Autodesk Fusion 360 part; units mm, degrees
note: some values were not read from the file. Set by a fixed rule: which sketch regions a step uses.
(part 2 of 3)
  line L698 (-202, 109) -> (-202, 113)
  arc A249 (-204, 107) -> (-202, 109) centre (-204, 109) ccw
  line L699 (-204, 107) -> (-241, 107)
  arc A250 (-241, 107) -> (-243, 105) centre (-241, 105) ccw
  line L700 (-243, 105) -> (-243, 99)
  arc A251 (-245, 97) -> (-243, 99) centre (-245, 99) ccw
  line L701 (-245, 97) -> (-267, 97)
  arc A252 (-332, 126.0001) -> (-330, 124.0001) centre (-330, 126.0001) ccw
  line L702 (-332, 126.0001) -> (-332, 135)
  line L703 (-332, 135) -> (-337, 135)
  line L704 (-337, 135) -> (-337, 133.0001)
  arc A253 (-339, 131.0001) -> (-337, 133.0001) centre (-339, 133.0001) ccw
  arc A254 (-358, 131.0001) -> (-362, 127) centre (-358, 127.0001) ccw
  line L705 (-362, 123) -> (-362, 127)
  arc A255 (-362, 123) -> (-358, 119.0001) centre (-358, 123.0001) ccw
  arc A256 (-337, 117) -> (-339, 119) centre (-339, 117) ccw
  line L706 (-337, 117) -> (-337, 115)
  line L707 (-337, 115) -> (-334, 115)
  arc A257 (-332, 113) -> (-334, 115) centre (-334, 113) ccw
  line L708 (-332, 109) -> (-332, 113)
  arc A258 (-332, 109) -> (-330, 107) centre (-330, 109) ccw
  line L709 (-330, 107) -> (-287, 107)
  arc A259 (-285, 105) -> (-287, 107) centre (-287, 105) ccw
  line L710 (-285, 105) -> (-285, 99)
  arc A260 (-285, 99) -> (-283, 97) centre (-283, 99) ccw
  line L711 (-283, 97) -> (-267, 97)
  line L712 (-267, 124) -> (-330, 124.0001)
  line L713 (-327, 5) -> (-327, 10)
  line L714 (-327, 10) -> (-307, 10)
  arc A261 (-223, 3) -> (-225, 5) centre (-225, 3) ccw
  line L715 (-225, 5) -> (-227, 5)
  line L716 (-227, 5) -> (-227, 10)
  line L717 (-207, 10) -> (-227, 10)
  line L718 (-207, 5) -> (-207, 10)
  line L719 (-207, 5) -> (-209.0021, 5)
  arc A262 (-209.0021, 5) -> (-211.0021, 2.9998) centre (-209.0021, 3) ccw
  line L720 (-211, -15.9146) -> (-211.0021, 2.9998)
  arc A263 (-215, -19.9102) -> (-211, -15.9146) centre (-215, -15.9102) ccw
  line L721 (-219, -19.9102) -> (-215, -19.9102)
  arc A264 (-223, -15.9116) -> (-219, -19.9102) centre (-219, -15.9102) ccw
  line L722 (-223, -15.9116) -> (-223, 3)
  line L723 (-225, 145) -> (-227, 145)
  line L724 (-227, 145) -> (-227, 140)
  line L725 (-207, 140) -> (-227, 140)
  line L726 (-207, 145) -> (-207, 140)
  line L727 (-207, 145) -> (-209.0021, 145)
  arc A265 (-211.0021, 147.0002) -> (-209.0021, 145) centre (-209.0021, 147) ccw
  line L728 (-211.0007, 166.0733) -> (-211.0021, 147.0002)
  arc A266 (-211.0007, 166.0733) -> (-215, 170) centre (-215, 166) ccw
  line L729 (-219, 170) -> (-215, 170)
  arc A267 (-219, 170) -> (-223, 166.0009) centre (-219, 166) ccw
  line L730 (-223, 166.0009) -> (-223, 147)
  arc A268 (-225, 145) -> (-223, 147) centre (-225, 147) ccw
  arc A269 (-311, 147) -> (-309, 145) centre (-309, 147) ccw
  line L731 (-309, 145) -> (-307, 145)
  line L732 (-307, 145) -> (-307, 140)
  line L733 (-327, 140) -> (-307, 140)
  line L734 (-327, 145) -> (-327, 140)
  line L735 (-327, 145) -> (-324.9979, 145)
  arc A270 (-324.9979, 145) -> (-322.9979, 147.0002) centre (-324.9979, 147) ccw
  line L736 (-322.9993, 165.9261) -> (-322.9979, 147.0002)
  arc A271 (-319, 170) -> (-322.9993, 165.9261) centre (-319, 166) ccw
  line L737 (-315, 170) -> (-319, 170)
  arc A272 (-311, 166.0009) -> (-315, 170) centre (-315, 166) ccw
  line L738 (-311, 166.0009) -> (-311, 147)
  circle A273 centre (43.5, 122.75) radius 3
  circle A274 centre (58.5, 122.75) radius 3
  circle A275 centre (73.5, 122.75) radius 3
  circle A276 centre (73.5, 27.25) radius 3
  arc A277 (79.466, 30.6504) -> (82, 35) centre (77, 35) ccw
  circle A278 centre (43.5, 17.25) radius 2.5
  circle A279 centre (58.5, 17.25) radius 2.5
  circle A280 centre (73.5, 132.75) radius 2.5
  circle A281 centre (58.5, 132.75) radius 2.5
  circle A282 centre (43.5, 132.75) radius 2.5
  line L739 (35, 5) -> (35, 10)
  line L740 (57.5, 5) -> (35, 5)
  line L741 (57.5, 10) -> (35, 10)
  line L742 (57.5, 5) -> (80, 5)
  line L743 (80, 5) -> (80, 10)
  line L744 (80, 10) -> (57.5, 10)
  line L745 (-10, -124) -> (-10, -114)
  line L746 (-10, -59) -> (-10, -69)
  line L747 (-13, -74) -> (-12, -74)
  line L748 (-12, -109) -> (-13, -109)
  line L749 (-15, -117) -> (-15, -114)
  arc A283 (-13, -109) -> (-14.3301, -109.5064) centre (-13, -111) ccw
  arc A284 (-12, -109) -> (-10, -107) centre (-12, -107) ccw
  arc A285 (-10, -76) -> (-12, -74) centre (-12, -76) ccw
  line L750 (-10, -76) -> (-10, -80.6987)
  line L751 (-10, -88.0192) -> (-10, -98.0192)
  arc A286 (-15, -72) -> (-14.9997, -72.0383) centre (-13, -72) ccw
  arc A287 (-14.3301, -73.4936) -> (-13, -74) centre (-13, -72) ccw
  line L752 (-15, -72) -> (-15, -67)
  line L753 (-135.6699, -107.8397) -> (-140, -105.3397)
  line L754 (-135.6699, -109.5064) -> (-135.6699, -107.8397)
  arc A288 (-135.6699, -109.5064) -> (-137, -109) centre (-137, -111) ccw
  line L755 (-138, -109) -> (-137, -109)
  line L756 (-140, -105.3398) -> (-140, -107)
  arc A289 (-140, -107) -> (-138, -109) centre (-138, -107) ccw
  line L757 (-139.9897, -75.7973) -> (-140, -80.6987)
  line L758 (-140, -80.6987) -> (-135.6699, -78.1987)
  arc A290 (-137, -74) -> (-135.6699, -73.4936) centre (-137, -72) ccw
  line L759 (-137, -74) -> (-138, -74)
  arc A291 (-138, -74) -> (-140, -76) centre (-138, -76) ccw
  line L760 (-140, -76) -> (-140, -80.6987)
  line L761 (-135.6699, -78.1987) -> (-135.6699, -73.4936)
  arc A292 (-133, -64) -> (-135, -66) centre (-133, -66) ccw
  line L762 (-133, -64) -> (-132, -64)
  arc A293 (-132, -64) -> (-131.6546, -63.9699) centre (-132, -62) ccw
  line L763 (-130.6699, -64.5385) -> (-131.6546, -63.9699)
  line L764 (-130.6699, -69.5385) -> (-130.6699, -64.5385)
  line L765 (-135, -72.0385) -> (-130.6699, -69.5385)
  line L766 (-135.0004, -72.0383) -> (-135, -72.0385)
  arc A294 (-135.0004, -72.0383) -> (-135, -72) centre (-137, -72) ccw
  line L767 (-135, -67) -> (-135, -66)
  line L768 (-135, -72) -> (-135, -67)
  line L769 (-90, -124) -> (-90, -129)
  line L770 (-90, -124) -> (-115, -124)
  line L771 (-115, -124) -> (-115, -129)
  line L772 (-115, -129) -> (-135, -129)
  line L773 (-135, -124) -> (-140, -124)
  line L774 (-140, -124) -> (-140, -114)
  line L775 (-145, -114) -> (-140, -114)
  line L776 (-145, -69) -> (-145, -114)
  line L777 (-140, -69) -> (-145, -69)
  line L778 (-140, -59) -> (-140, -69)
  line L779 (-140, -59) -> (-135, -59)
  line L780 (-135, -54) -> (-135, -59)
  line L781 (-135, -49) -> (-135, -54)
  arc A295 (-131.8566, -44.3575) -> (-135, -49) centre (-130, -49) ccw
  arc A296 (-115, -49) -> (-118.1434, -44.3575) centre (-120, -49) ccw
  line L782 (-115, -54) -> (-115, -49)
  line L783 (-115, -59) -> (-115, -54)
  line L784 (-115, -59) -> (-94.5, -59)
  line L785 (-94.5, -59) -> (-94.5, -39)
  arc A297 (-89.5, -34) -> (-94.5, -39) centre (-89.5, -39) ccw
  line L786 (-135, -129) -> (-135, -124)
  line L787 (-90, -129) -> (-60, -129)
  circle A298 centre (-85, -48) radius 4.075
  circle A299 centre (-275.5, -32.5) radius 4.075
  line L788 (-209.5, -99.5) -> (-209.5, -103.5)
  line L789 (-207.5, -105.5) -> (-206, -105.5)
  line L790 (-204, -103.5) -> (-204, -99.5)
  line L791 (-206, -97.5) -> (-207.5, -97.5)
  arc A300 (-207.5, -97.5) -> (-209.5, -99.5) centre (-207.5, -99.5) ccw
  arc A301 (-204, -99.5) -> (-206, -97.5) centre (-206, -99.5) ccw
  arc A302 (-206, -105.5) -> (-204, -103.5) centre (-206, -103.5) ccw
  arc A303 (-209.5, -103.5) -> (-207.5, -105.5) centre (-207.5, -103.5) ccw
  arc A304 (-321.5, -99.5) -> (-323.5, -97.5) centre (-323.5, -99.5) ccw
  line L792 (-321.5, -99.5) -> (-321.5, -103.5)
  arc A305 (-323.5, -105.5) -> (-321.5, -103.5) centre (-323.5, -103.5) ccw
  line L793 (-323.5, -105.5) -> (-325, -105.5)
  arc A306 (-327, -103.5) -> (-325, -105.5) centre (-325, -103.5) ccw
  line L794 (-327, -103.5) -> (-327, -99.5)
  arc A307 (-325, -97.5) -> (-327, -99.5) centre (-325, -99.5) ccw
  line L795 (-325, -97.5) -> (-323.5, -97.5)
  arc A308 (41.7475, 118.6053) -> (45.2525, 118.6053) centre (43.5, 122.75) ccw
  line L796 (34, 119) -> (39.8003, 119)
  line L797 (47.1997, 119) -> (54.8003, 119)
  arc A309 (56.7475, 118.6053) -> (60.2525, 118.6053) centre (58.5, 122.75) ccw
  line L798 (62.1997, 119) -> (69.8003, 119)
  line L799 (77.1997, 119) -> (81, 119)
  arc A310 (71.7475, 118.6053) -> (75.2525, 118.6053) centre (73.5, 122.75) ccw
  arc A311 (41.7475, 118.6053) -> (39.8003, 119) centre (39.8003, 114) ccw
  arc A312 (47.1997, 119) -> (45.2525, 118.6053) centre (47.1997, 114) ccw
  arc A313 (56.7475, 118.6053) -> (54.8003, 119) centre (54.8003, 114) ccw
  arc A314 (62.1997, 119) -> (60.2525, 118.6053) centre (62.1997, 114) ccw
  arc A315 (71.7475, 118.6053) -> (69.8003, 119) centre (69.8003, 114) ccw
  arc A316 (77.1997, 119) -> (75.2525, 118.6053) centre (77.1997, 114) ccw
  line L800 (-82.0096, -106.5) -> (-77.9904, -106.5)
  line L801 (-72.0096, -106.5) -> (-67.9904, -106.5)
  arc A317 (-289.5, 21) -> (-291.5, 23) centre (-291.5, 21) ccw
  line L802 (-291.5, 23) -> (-327, 23)
  arc A318 (-327, 23) -> (-329, 21) centre (-327, 21) ccw
  line L803 (-329, 15) -> (-329, 21)
  arc A319 (-329, 15) -> (-327, 13) centre (-327, 15) ccw
  line L804 (-249.5, 23) -> (-284.5, 23)
  arc A320 (-284.5, 23) -> (-286.5, 21) centre (-284.5, 21) ccw
  arc A321 (-247.5, 21) -> (-249.5, 23) centre (-249.5, 21) ccw
  line L805 (-337, 108) -> (-337, 94.5)
  arc A322 (-337, 108) -> (-339, 110) centre (-339, 108) ccw
  line L806 (-339, 110) -> (-340, 110)
  arc A323 (-342, 112) -> (-340, 110) centre (-340, 112) ccw
  line L807 (-342, 112) -> (-342, 112.9999)
  arc A324 (-342, 112.9999) -> (-344, 114.9999) centre (-344, 112.9999) ccw
  arc A325 (-366, 122.9999) -> (-358, 114.9999) centre (-358, 122.9999) ccw
  line L808 (-366, 126.9998) -> (-366, 122.9999)
  arc A326 (-358, 134.9998) -> (-366, 126.9998) centre (-358, 126.9998) ccw
  arc A327 (-344, 134.9999) -> (-342, 136.9999) centre (-344, 136.9999) ccw
  line L809 (-342, 136.9999) -> (-342.0001, 145)
  arc A328 (-337, 150) -> (-342.0001, 145) centre (-337, 145) ccw
  line L810 (-337, 150) -> (-329, 150)
  arc A329 (-329, 150) -> (-327, 152) centre (-329, 152) ccw
  line L811 (-327, 166) -> (-327, 152)
  arc A330 (-319, 174) -> (-327, 166) centre (-319, 166) ccw
  line L812 (-315, 174) -> (-319, 174)
  arc A331 (-307, 166.0013) -> (-315, 174) centre (-315, 166) ccw
  line L813 (-307, 152) -> (-307, 166.0013)
  arc A332 (-307, 152) -> (-305, 150) centre (-305, 152) ccw
  line L814 (-305, 150) -> (-304, 150)
  arc A333 (-302, 148) -> (-304, 150) centre (-304, 148) ccw
  line L815 (-302, 147) -> (-302, 148)
  arc A334 (-302, 147) -> (-300, 145) centre (-300, 147) ccw
  line L816 (-300, 145) -> (-286.5, 145)
  line L817 (-247.5, 144.9999) -> (-233.9999, 144.9999)
  arc A335 (-233.9999, 144.9999) -> (-231.9997, 147.0001) centre (-233.9999, 147.0001) ccw
  line L818 (-231.9997, 147.0001) -> (-231.9997, 147.9994)
  arc A336 (-229.999, 150.0001) -> (-231.9997, 147.9994) centre (-229.999, 147.9994) ccw
  line L819 (-229, 150.0001) -> (-229.999, 150.0001)
  arc A337 (-229, 150.0001) -> (-227, 152.0001) centre (-229, 152.0001) ccw
  line L820 (-227, 152.0001) -> (-227, 166.002)
  arc A338 (-219, 174) -> (-227, 166.002) centre (-219, 166) ccw
  line L821 (-219, 174) -> (-215, 174)
  arc A339 (-207, 166) -> (-215, 174) centre (-215, 166) ccw
  line L822 (-207, 166) -> (-207, 152.0001)
  arc A340 (-207, 152.0001) -> (-205, 150.0001) centre (-205, 152.0001) ccw
  line L823 (-197, 150.0001) -> (-205, 150.0001)
  arc A341 (-192, 145.0001) -> (-197, 150.0001) centre (-197, 145.0001) ccw
  line L824 (-192, 145.0001) -> (-192, 136.9999)
  arc A342 (-192, 136.9999) -> (-190, 134.9999) centre (-190, 136.9999) ccw
  arc A343 (-168, 126.9998) -> (-175.9914, 134.9998) centre (-176, 126.9998) ccw
  line L825 (-168, 126.9998) -> (-168, 122.9999)
  arc A344 (-176, 114.9999) -> (-168, 122.9999) centre (-176, 122.9999) ccw
  arc A345 (-190, 114.9999) -> (-192, 112.9999) centre (-190, 112.9999) ccw
  line L826 (-192, 112) -> (-192, 112.9999)
  arc A346 (-194, 110) -> (-192, 112) centre (-194, 112) ccw
  line L827 (-195, 110) -> (-194, 110)
  arc A347 (-195, 110) -> (-197, 108) centre (-195, 108) ccw
  line L828 (-197, 108) -> (-197, 90)
  line L829 (-197, 90) -> (-202, 90)
  line L830 (-202, 90) -> (-202, 75)
  line L831 (-104, 5) -> (-86, 5)
  line L832 (-56, 5) -> (-38, 5)
  line L833 (-104, 145) -> (-86, 145)
  line L834 (-56, 145) -> (-38, 145)
  line L835 (-141, 90) -> (-141, 108)
  line L836 (-141, 60) -> (-141, 42)
  line L837 (-302, 8) -> (-291.5, 8)
  line L838 (-327, 13) -> (-306, 13)
  line L839 (-304, 11) -> (-304, 10)
  line L840 (-289.5, 21) -> (-289.5, 10)
  arc A348 (-304, 11) -> (-306, 13) centre (-306, 11) ccw
  arc A349 (-304, 10) -> (-302, 8) centre (-302, 10) ccw
  arc A350 (-291.5, 8) -> (-289.5, 10) centre (-291.5, 10) ccw
  arc A351 (-244.5001, 10) -> (-242.5001, 8) centre (-242.5001, 10) ccw
  line L841 (-232.0001, 7.9999) -> (-242.5001, 8)
  arc A352 (-232.0001, 7.9999) -> (-230.0001, 9.9999) centre (-232.0001, 9.9999) ccw
  line L842 (-230.0001, 10.9999) -> (-230.0001, 9.9999)
  arc A353 (-228.0001, 12.9999) -> (-230.0001, 10.9999) centre (-228.0001, 10.9999) ccw
  line L843 (-207.0001, 12.9999) -> (-228.0001, 12.9999)
  arc A354 (-207.0001, 12.9999) -> (-205.0001, 14.9999) centre (-207.0001, 14.9999) ccw
  line L844 (-205.0001, 14.9999) -> (-205.0001, 20.9999)
  arc A355 (-205.0001, 20.9999) -> (-207.0001, 22.9999) centre (-207.0001, 20.9999) ccw
  line L845 (-242.4962, 23) -> (-207.0001, 22.9999)
  arc A356 (-242.4962, 23) -> (-244.5001, 21) centre (-242.5001, 21) ccw
  line L846 (-244.5001, 21) -> (-244.5001, 10)
  line L847 (-329, 135) -> (-329, 129)
  arc A357 (-327, 137) -> (-329, 135) centre (-327, 135) ccw
  line L848 (-327, 137) -> (-306, 137)
  arc A358 (-306, 137) -> (-304, 139) centre (-306, 139) ccw
  line L849 (-304, 139) -> (-304, 140)
  arc A359 (-302, 142) -> (-304, 140) centre (-302, 140) ccw
  line L850 (-302, 142) -> (-291.5, 142)
  arc A360 (-289.5, 140) -> (-291.5, 142) centre (-291.5, 140) ccw
  line L851 (-289.5, 129) -> (-289.5, 140)
  arc A361 (-291.5, 127) -> (-289.5, 129) centre (-291.5, 129) ccw
  line L852 (-291.5, 127) -> (-327, 127)
  arc A362 (-329, 129) -> (-327, 127) centre (-327, 129) ccw
  arc A363 (-207.0001, 127.0001) -> (-205.0001, 129.0001) centre (-207.0001, 129.0001) ccw
  line L853 (-205.0001, 135.0001) -> (-205.0001, 129.0001)
  arc A364 (-205.0001, 135.0001) -> (-207.0001, 137.0001) centre (-207.0001, 135.0001) ccw
  line L854 (-207.0001, 137.0001) -> (-228.0001, 137.0001)
  arc A365 (-230.0001, 139.0001) -> (-228.0001, 137.0001) centre (-228.0001, 139.0001) ccw
  line L855 (-230.0001, 139.0001) -> (-230.0001, 140.0001)
  arc A366 (-230.0001, 140.0001) -> (-232.0001, 142.0001) centre (-232.0001, 140.0001) ccw
  line L856 (-232.0001, 142.0001) -> (-242.5001, 142)
  arc A367 (-242.5001, 142) -> (-244.5001, 140) centre (-242.5001, 140) ccw
  line L857 (-244.5001, 129) -> (-244.5001, 140)
  arc A368 (-244.5001, 129) -> (-242.4962, 127) centre (-242.5001, 129) ccw
  line L858 (-242.4962, 127) -> (-207.0001, 127.0001)
  line L859 (-200.5, -98.5) -> (-200.5, -53.5)
  line L860 (-335.5, -76) -> (-335.5, -53.5)
  line L861 (-335.5, -76) -> (-335.5, -98.5)
  line L862 (-335.5, -98.5) -> (-330.5, -98.5)
  line L863 (-330.5, -98.5) -> (-330.5, -53.5)
  line L864 (-335.5, -53.5) -> (-330.5, -53.5)
  line L865 (-136, 10) -> (-141, 10)
  line L866 (-141, 5) -> (-136, 5)
  line L867 (-136, 5) -> (-136, 10)
  line L868 (-141, 10) -> (-141, 5)
  line L869 (-1, 5) -> (-6, 5)
  line L870 (-6, 5) -> (-6, 10)
  line L871 (-6, 10) -> (-1, 10)
  line L872 (-1, 10) -> (-1, 5)
  line L873 (-136, 145) -> (-136, 140)
  line L874 (-136, 140) -> (-141, 140)
  line L875 (-141, 140) -> (-141, 145)
  line L876 (-141, 145) -> (-136, 145)
  line L877 (-6, 145) -> (-6, 140)
  line L878 (-6, 140) -> (-1, 140)
  line L879 (-1, 140) -> (-1, 145)
  line L880 (-1, 145) -> (-6, 145)
  circle A369 centre (-125, -40) radius 2.5
  arc A370 (-119.3006, -41.8753) -> (-130.6994, -41.8753) centre (-125, -40) ccw
  arc A371 (-119.3006, -41.8753) -> (-118.1434, -44.3575) centre (-117.4008, -42.5004) ccw
  arc A372 (-131.8566, -44.3575) -> (-130.6994, -41.8753) centre (-132.5992, -42.5004) ccw
  arc A373 (-15, -49) -> (-18.1435, -44.3575) centre (-20, -49) ccw
  arc A374 (-19.3006, -41.8753) -> (-18.1435, -44.3575) centre (-17.4008, -42.5004) ccw
  arc A375 (-19.3006, -41.8753) -> (-30.6994, -41.8753) centre (-25, -40) ccw
  circle A376 centre (-25, -40) radius 2.5
  arc A377 (-31.8566, -44.3575) -> (-35, -49) centre (-30, -49) ccw
  arc A378 (-31.8566, -44.3575) -> (-30.6994, -41.8753) centre (-32.5992, -42.5004) ccw
  line L881 (-286.5, 5) -> (-286.5, 11)
  line L882 (-284.5, 13) -> (-249.5, 13)
  line L883 (-247.5, 11) -> (-247.5, 5.0001)
  arc A379 (-249.5, 16) -> (-247.5, 18) centre (-249.5, 18) ccw
  line L884 (-249.5, 16) -> (-284.5, 16)
  arc A380 (-286.5, 18) -> (-284.5, 16) centre (-284.5, 18) ccw
  arc A381 (-284.5, 13) -> (-286.5, 11) centre (-284.5, 11) ccw
  arc A382 (-247.5, 11) -> (-249.5, 13) centre (-249.5, 11) ccw
  line L885 (-286.5, 18) -> (-286.5, 21)
  line L886 (-247.5, 21) -> (-247.5, 18)
  line L887 (-284.5, 137) -> (-249.5, 137)
  arc A383 (-284.5, 134) -> (-286.5, 132) centre (-284.5, 132) ccw
  line L888 (-286.5, 132) -> (-286.5, 129)
  arc A384 (-286.5, 129) -> (-284.5, 127) centre (-284.5, 129) ccw
  line L889 (-249.5, 127) -> (-284.5, 127)
  arc A385 (-249.5, 127) -> (-247.5, 129) centre (-249.5, 129) ccw
  line L890 (-247.5, 129) -> (-247.5, 132)
  arc A386 (-247.5, 132) -> (-249.5, 134) centre (-249.5, 132) ccw
  line L891 (-249.5, 134) -> (-284.5, 134)
  arc A387 (-286.5, 139) -> (-284.5, 137) centre (-284.5, 139) ccw
  line L892 (-286.5, 145) -> (-286.5, 139)
  line L893 (-247.5, 139) -> (-247.5, 144.9999)
  arc A388 (-249.5, 137) -> (-247.5, 139) centre (-249.5, 139) ccw
  line L894 (-337, 94.5) -> (-331, 94.5)
  line L895 (-337, 55.5) -> (-331, 55.5)
  line L896 (-329, 92.5) -> (-329, 57.5)
  arc A389 (-329, 92.5) -> (-331, 94.5) centre (-331, 92.5) ccw
  arc A390 (-331, 55.5) -> (-329, 57.5) centre (-331, 57.5) ccw
  arc A391 (76.1918, 30.8561) -> (70.8974, 30.9211) centre (73.5, 27.25) ccw
  line L897 (38, 30) -> (68.0057, 30)
  arc A392 (68.0057, 30) -> (70.8974, 30.9211) centre (68.0057, 35) ccw
  arc A393 (76.1918, 30.8561) -> (79.466, 30.6504) centre (77.9864, 33.2602) ccw
  line L898 (-195, 18.9999) -> (-176, 18.9999)
  line L899 (-190, 15.0001) -> (-175.9914, 15.0002)
  line L900 (-190, 35.0001) -> (-176, 35.0001)
  line L901 (-195, 31) -> (-176, 30.9999)
  line L902 (-195, 119) -> (-176, 119.0001)
  line L903 (-190, 114.9999) -> (-176, 114.9999)
  line L904 (-195, 131.0001) -> (-176, 131.0001)
  line L905 (-190, 134.9999) -> (-175.9914, 134.9998)
  line L906 (-358, 134.9998) -> (-344, 134.9999)
  line L907 (-358, 131.0001) -> (-339, 131.0001)
  line L908 (-358, 119.0001) -> (-339, 119)
  line L909 (-358, 114.9999) -> (-344, 114.9999)
  line L910 (-358, 35.0001) -> (-344, 35.0001)
  line L911 (-358, 30.9999) -> (-339, 31)
  line L912 (-358, 18.9999) -> (-339, 18.9999)
  line L913 (-358, 15.0002) -> (-344, 15.0001)
  circle A394 centre (-240, 91) radius 1.5
  circle A395 centre (-208, 91) radius 1.5
  circle A396 centre (-240, 59) radius 1.5
  circle A397 centre (-208, 59) radius 1.5
  line L914 (-240, 65.3246) -> (-240, 84.6754)
  line L915 (-214.3246, 59) -> (-233.6754, 59)
  line L916 (-238.5, 59) -> (-240, 59)
  arc A398 (-236.386, 60.7143) -> (-238.2857, 62.614) centre (-240, 59) ccw
  arc A399 (-238.2857, 87.386) -> (-236.386, 89.2857) centre (-240, 91) ccw
  arc A400 (-211.614, 89.2857) -> (-209.7143, 87.386) centre (-208, 91) ccw
  line L917 (-233.6754, 91) -> (-214.3246, 91)
  line L918 (-208, 84.6754) -> (-208, 65.3246)
  arc A401 (-209.7143, 62.614) -> (-211.614, 60.7143) centre (-208, 59) ccw
  arc A402 (-238.2857, 87.386) -> (-240, 84.6754) centre (-237, 84.6754) ccw
  arc A403 (-233.6754, 91) -> (-236.386, 89.2857) centre (-233.6754, 88) ccw
  arc A404 (-240, 65.3246) -> (-238.2857, 62.614) centre (-237, 65.3246) ccw
  arc A405 (-236.386, 60.7143) -> (-233.6754, 59) centre (-233.6754, 62) ccw
  arc A406 (-214.3246, 59) -> (-211.614, 60.7143) centre (-214.3246, 62) ccw
  arc A407 (-209.7143, 62.614) -> (-208, 65.3246) centre (-211, 65.3246) ccw
  arc A408 (-208, 84.6754) -> (-209.7143, 87.386) centre (-211, 84.6754) ccw
  arc A409 (-211.614, 89.2857) -> (-214.3246, 91) centre (-214.3246, 88) ccw
  circle A410 centre (30, -80) radius 1
  circle A411 centre (30, -108) radius 1
  arc A412 (31.1111, -82.2395) -> (32.2395, -81.1111) centre (30, -80) ccw
  line L919 (30, -103.9689) -> (30, -84.0311)
  line L920 (34.0311, -80) -> (44, -80)
  arc A413 (30, -103.9689) -> (31.1111, -105.7605) centre (32, -103.9689) ccw
  arc A414 (34.0311, -80) -> (32.2395, -81.1111) centre (34.0311, -82) ccw
  arc A415 (31.1111, -82.2395) -> (30, -84.0311) centre (32, -84.0311) ccw
  line L921 (19.75, -89.25) -> (19.75, -95.75)
  line L922 (22.25, -89.2502) -> (22.25, -95.75)
  arc A416 (22.25, -89.2502) -> (19.75, -89.25) centre (21, -89.25) ccw
  arc A417 (19.75, -95.75) -> (22.25, -95.75) centre (21, -95.75) ccw
  line L923 (-75, -55) -> (-90, -55)
  line L924 (-92, -57) -> (-92, -103)
  line L925 (-90, -105) -> (-60, -105)
  line L926 (-58, -103) -> (-58, -57)
  line L927 (-60, -55) -> (-75, -55)
  arc A418 (22.25, -107.25) -> (19.75, -107.25) centre (21, -107.25) ccw
  line L928 (19.75, -113.75) -> (19.75, -107.25)
  arc A419 (19.75, -113.75) -> (22.25, -113.7498) centre (21, -113.75) ccw
  line L929 (22.25, -113.7498) -> (22.25, -107.25)
  line L930 (-87.9002, -106.5521) -> (-92.1651, -106.5898)
  line L931 (-62.0096, -106.5) -> (-57.9904, -106.5)
  arc A420 (-90, -55) -> (-92, -57) centre (-90, -57) ccw
  arc A421 (-58, -57) -> (-60, -55) centre (-60, -57) ccw
  arc A422 (-60, -105) -> (-58, -103) centre (-60, -103) ccw
  arc A423 (-92, -103) -> (-90, -105) centre (-90, -103) ccw
  line L932 (-89.5, -34) -> (-60.5, -34)
  arc A424 (32.5, -108) -> (31.1111, -105.7605) centre (30, -108) ccw
  line L933 (21, -99.7811) -> (21, -103.2189)
  line L934 (32.5, -108) -> (32.5, -110.7498)
  line L935 (29.5, -113.7498) -> (25.0312, -113.7498)
  line L936 (18.5, -113.7498) -> (18.5, -107.25)
  line L937 (18.5, -95.75) -> (18.5, -89.25)
  arc A425 (18.5, -113.7498) -> (23.2396, -114.861) centre (21, -113.75) ccw
  arc A426 (19.8889, -105.0105) -> (18.5, -107.25) centre (21, -107.25) ccw
  arc A427 (18.5, -95.75) -> (19.8889, -97.9895) centre (21, -95.75) ccw
  line L938 (30, -77.5) -> (44, -77.5)
  arc A428 (31.1111, -82.2395) -> (32.2395, -81.1111) centre (30, -80) ccw
  arc A429 (30, -77.5) -> (27.5, -80) centre (30, -80) ccw
  arc A430 (21, -99.7811) -> (19.8889, -97.9895) centre (19, -99.7811) ccw
  arc A431 (19.8889, -105.0105) -> (21, -103.2189) centre (19, -103.2189) ccw
  arc A432 (25.0312, -113.7498) -> (23.2396, -114.861) centre (25.0312, -115.7498) ccw
  arc A433 (29.5, -113.7498) -> (32.5, -110.7498) centre (29.5, -110.7498) ccw
  circle A434 centre (58, -108) radius 1
  line L939 (68.25, -113.75) -> (68.25, -107.25)
  arc A435 (65.75, -113.7498) -> (68.25, -113.75) centre (67, -113.75) ccw
  arc A436 (68.25, -107.25) -> (65.75, -107.25) centre (67, -107.25) ccw
  line L940 (65.75, -113.7498) -> (65.75, -107.25)
  arc A437 (65.75, -95.75) -> (68.25, -95.75) centre (67, -95.75) ccw
  line L941 (68.25, -89.25) -> (68.25, -95.75)
  arc A438 (68.25, -89.25) -> (65.75, -89.2502) centre (67, -89.25) ccw
  line L942 (65.75, -89.2502) -> (65.75, -95.75)
  circle A439 centre (58, -80) radius 1
  line L943 (-55.25, -93.75) -> (-48.75, -93.75)
  line L944 (-55.25, -96.25) -> (-48.75, -96.25)
  arc A440 (-55.25, -93.75) -> (-55.25, -96.25) centre (-55.25, -95) ccw
  arc A441 (-48.75, -96.25) -> (-48.75, -93.75) centre (-48.75, -95) ccw
  line L945 (-55.25, -75.75) -> (-48.75, -75.75)
  arc A442 (-55.25, -75.75) -> (-55.25, -78.25) centre (-55.25, -77) ccw
  line L946 (-55.25, -78.25) -> (-48.75, -78.25)
  arc A443 (-48.75, -78.25) -> (-48.75, -75.75) centre (-48.75, -77) ccw
  line L947 (-94.75, -93.75) -> (-101.25, -93.75)
  arc A444 (-94.75, -96.25) -> (-94.75, -93.75) centre (-94.75, -95) ccw
  line L948 (-94.75, -96.25) -> (-101.25, -96.25)
  arc A445 (-101.25, -93.75) -> (-101.25, -96.25) centre (-101.25, -95) ccw
  line L949 (-94.75, -75.75) -> (-101.25, -75.75)
  arc A446 (-94.75, -78.25) -> (-94.75, -75.75) centre (-94.75, -77) ccw
  arc A447 (-101.25, -75.75) -> (-101.25, -78.25) centre (-101.25, -77) ccw
  line L950 (-94.75, -78.25) -> (-101.25, -78.25)
  line L951 (27.5, -80) -> (27.5, -87)
  line L952 (25.5, -89) -> (24.8971, -89)
  arc A448 (23.1651, -88) -> (18.5, -89.25) centre (21, -89.25) ccw
  arc A449 (23.1651, -88) -> (24.8971, -89) centre (24.8971, -87) ccw
  arc A450 (25.5, -89) -> (27.5, -87) centre (25.5, -87) ccw
  arc A451 (58, -84.0311) -> (56.8889, -82.2395) centre (56, -84.0311) ccw
  line L953 (58, -103.9689) -> (58, -84.0311)
  arc A452 (56.8889, -105.7605) -> (58, -103.9689) centre (56, -103.9689) ccw
  arc A453 (56.8889, -105.7605) -> (55.5, -108) centre (58, -108) ccw
  line L954 (55.5, -108) -> (55.5, -110.7498)
  arc A454 (55.5, -110.7498) -> (58.5, -113.7498) centre (58.5, -110.7498) ccw
  line L955 (58.5, -113.7498) -> (62.9688, -113.7498)
  arc A455 (64.7604, -114.861) -> (62.9688, -113.7498) centre (62.9688, -115.7498) ccw
  arc A456 (64.7604, -114.861) -> (69.5, -113.7498) centre (67, -113.75) ccw
  line L956 (69.5, -113.7498) -> (69.5, -107.25)
  arc A457 (69.5, -107.25) -> (68.1111, -105.0105) centre (67, -107.25) ccw
  arc A458 (67, -103.2189) -> (68.1111, -105.0105) centre (69, -103.2189) ccw
  line L957 (67, -99.7811) -> (67, -103.2189)
  arc A459 (68.1111, -97.9895) -> (67, -99.7811) centre (69, -99.7811) ccw
  arc A460 (68.1111, -97.9895) -> (69.5, -95.75) centre (67, -95.75) ccw
  line L958 (69.5, -95.75) -> (69.5, -89.25)
  arc A461 (69.5, -89.25) -> (64.8349, -88) centre (67, -89.25) ccw
  arc A462 (63.1029, -89) -> (64.8349, -88) centre (63.1029, -87) ccw
  line L959 (62.5, -89) -> (63.1029, -89)
  arc A463 (60.5, -87) -> (62.5, -89) centre (62.5, -87) ccw
  line L960 (60.5, -80) -> (60.5, -87)
  arc A464 (60.5, -80) -> (58, -77.5) centre (58, -80) ccw
  line L961 (58, -77.5) -> (44, -77.5)
  arc A465 (55.7605, -81.1111) -> (56.8889, -82.2395) centre (58, -80) ccw
  arc A466 (55.7605, -81.1111) -> (53.9689, -80) centre (53.9689, -82) ccw
  line L962 (53.9689, -80) -> (44, -80)
  line L963 (-280.5, -89.5) -> (-250.5, -89.5)
  arc A467 (-250.5, -89.5) -> (-248.5, -87.5) centre (-250.5, -87.5) ccw
  line L964 (-248.5, -87.5) -> (-248.5, -41.5)
  arc A468 (-248.5, -41.5) -> (-250.5, -39.5) centre (-250.5, -41.5) ccw
  line L965 (-250.5, -39.5) -> (-265.5, -39.5)
  line L966 (-265.5, -39.5) -> (-280.5, -39.5)
  arc A469 (-280.5, -39.5) -> (-282.5, -41.5) centre (-280.5, -41.5) ccw
  line L967 (-282.5, -41.5) -> (-282.5, -87.5)
  arc A470 (-282.5, -87.5) -> (-280.5, -89.5) centre (-280.5, -87.5) ccw
  arc A471 (-291.75, -78.25) -> (-291.75, -80.75) centre (-291.75, -79.5) ccw
  line L968 (-285.25, -78.25) -> (-291.75, -78.25)
  arc A472 (-285.25, -80.75) -> (-285.25, -78.25) centre (-285.25, -79.5) ccw
  line L969 (-285.25, -80.75) -> (-291.75, -80.75)
  arc A473 (-291.75, -60.25) -> (-291.75, -62.75) centre (-291.75, -61.5) ccw
  line L970 (-285.25, -60.25) -> (-291.75, -60.25)
  arc A474 (-285.25, -62.75) -> (-285.25, -60.25) centre (-285.25, -61.5) ccw
  line L971 (-285.25, -62.75) -> (-291.75, -62.75)
  line L972 (-245.75, -60.25) -> (-239.25, -60.25)
  arc A475 (-245.75, -60.25) -> (-245.75, -62.75) centre (-245.75, -61.5) ccw
  arc A476 (-239.25, -62.75) -> (-239.25, -60.25) centre (-239.25, -61.5) ccw
  line L973 (-245.75, -62.75) -> (-239.25, -62.75)
  line L974 (-245.75, -78.25) -> (-239.25, -78.25)
  arc A477 (-245.75, -78.25) -> (-245.75, -80.75) centre (-245.75, -79.5) ccw
  arc A478 (-239.25, -80.75) -> (-239.25, -78.25) centre (-239.25, -79.5) ccw
  line L975 (-245.75, -80.75) -> (-239.25, -80.75)
  arc A479 (-232.386, -85.2857) -> (-229.6754, -87) centre (-229.6754, -84) ccw
  arc A480 (-232.386, -85.2857) -> (-234.2857, -83.386) centre (-236, -87) ccw
  arc A481 (-236, -80.6754) -> (-234.2857, -83.386) centre (-233, -80.6754) ccw
  line L976 (-236, -80.6754) -> (-236, -61.3246)
  arc A482 (-234.2857, -58.614) -> (-236, -61.3246) centre (-233, -61.3246) ccw
  arc A483 (-234.2857, -58.614) -> (-232.386, -56.7143) centre (-236, -55) ccw
  arc A484 (-229.6754, -55) -> (-232.386, -56.7143) centre (-229.6754, -58) ccw
  line L977 (-229.6754, -55) -> (-210.3246, -55)
  arc A485 (-207.614, -56.7143) -> (-210.3246, -55) centre (-210.3246, -58) ccw
  arc A486 (-207.614, -56.7143) -> (-205.7143, -58.614) centre (-204, -55) ccw
  arc A487 (-204, -61.3246) -> (-205.7143, -58.614) centre (-207, -61.3246) ccw
  line L978 (-204, -61.3246) -> (-204, -80.6754)
  arc A488 (-205.7143, -83.386) -> (-204, -80.6754) centre (-207, -80.6754) ccw
  arc A489 (-205.7143, -83.386) -> (-207.614, -85.2857) centre (-204, -87) ccw
  arc A490 (-210.3246, -87) -> (-207.614, -85.2857) centre (-210.3246, -84) ccw
  line L979 (-210.3246, -87) -> (-229.6754, -87)
  circle A491 centre (-236, -87) radius 1.5
  circle A492 centre (-236, -55) radius 1.5
  circle A493 centre (-204, -55) radius 1.5
  circle A494 centre (-204, -87) radius 1.5
  circle A495 centre (-295, -87) radius 1.5
  arc A496 (-301.3246, -87) -> (-298.614, -85.2857) centre (-301.3246, -84) ccw
  arc A497 (-296.7143, -83.386) -> (-298.614, -85.2857) centre (-295, -87) ccw
  arc A498 (-296.7143, -83.386) -> (-295, -80.6754) centre (-298, -80.6754) ccw
  line L980 (-295, -80.6754) -> (-295, -61.3246)
  arc A499 (-295, -61.3246) -> (-296.7143, -58.614) centre (-298, -61.3246) ccw
  arc A500 (-298.614, -56.7143) -> (-296.7143, -58.614) centre (-295, -55) ccw
  arc A501 (-298.614, -56.7143) -> (-301.3246, -55) centre (-301.3246, -58) ccw
  line L981 (-301.3246, -55) -> (-320.6755, -55)
  arc A502 (-320.6755, -55) -> (-323.386, -56.7143) centre (-320.6755, -58) ccw
  arc A503 (-325.2857, -58.614) -> (-323.386, -56.7143) centre (-327, -55) ccw
  arc A504 (-325.2857, -58.614) -> (-327, -61.3246) centre (-324, -61.3246) ccw
  line L982 (-327, -61.3246) -> (-327, -80.6754)
  arc A505 (-327, -80.6754) -> (-325.2857, -83.386) centre (-324, -80.6754) ccw
  arc A506 (-323.386, -85.2857) -> (-325.2857, -83.386) centre (-327, -87) ccw
  arc A507 (-323.386, -85.2857) -> (-320.6755, -87) centre (-320.6755, -84) ccw
  line L983 (-320.6755, -87) -> (-301.3246, -87)
  circle A508 centre (-295, -55) radius 1.5
  circle A509 centre (-327, -55) radius 1.5
  circle A510 centre (-327, -87) radius 1.5
  line L984 (-307, -93) -> (-224, -93)
  line L985 (-221, -96) -> (-221, -102)
  line L986 (-224, -105) -> (-307, -105)
  line L987 (-310, -102) -> (-310, -96)
  arc A511 (-307, -93) -> (-310, -96) centre (-307, -96) ccw
  arc A512 (-310, -102) -> (-307, -105) centre (-307, -102) ccw
  arc A513 (-224, -105) -> (-221, -102) centre (-224, -102) ccw
  arc A514 (-221, -96) -> (-224, -93) centre (-224, -96) ccw
  point P0 (-192, 0)
  point P1 (-75, -119)
  point P2 (-80, -110.3397)
  point P3 (-120, -58.3782)
  point P4 (-75, -119)
  point P5 (-75.0001, -119)
  point P6 (-75, -119)
  point P7 (-75, -119)
  point P8 (-75, -119)
  point P9 (-70, -110.3397)
  point P10 (-75, -119)
  point P11 (-75, -119)
  point P12 (-30, -58.3782)
  point P13 (35, -40)
  point P14 (35, -35)
  point P15 (-92, -55)
  point P16 (-92, -105)
  point P17 (-58, -105)
  point P18 (44, -92.3923)
  dimension "d35" = 5
  dimension "d36" = 5
  dimension "d40" = 5
  dimension "d41" = 2
  dimension "d67" = 5
  dimension "d68" = 5
  dimension "d69" = 2
  dimension "d89" = 5
  dimension "d94" = 5
  dimension "d112" = 2.5
  dimension "d113" = 2.5
  dimension "d116" = 2.5
  dimension "d369" = 2
  dimension "d426" = 3
  dimension "d427" = 3
  dimension "d429" = 3
  dimension "d466" = 8
  dimension "d474" = 3
  dimension "d508" = 3
  dimension "d524" = 8
  dimension "d525" = 8
  dimension "d526" = 4
  dimension "d527" = 2
  dimension "d528" = 1
  dimension "d529" = 2
  dimension "d532" = 14
  dimension "d533" = 14
  dimension "d534" = 14
  dimension "d535" = 14
  dimension "d545" = 2
  dimension "d546" = 8
  dimension "d555" = 3
  dimension "d557" = 1
  dimension "d579" = 1
  dimension "d589" = 10
  dimension "d591" = 5
  dimension "d592" = 5
  dimension "d593" = 5
  dimension "d594" = 5
  dimension "d604" = 5
  dimension "d605" = 2
  dimension "d643" = 1
  dimension "d648" = 2
  dimension "d652" = 2
  dimension "d654" = 5
  dimension "d655" = 5
  dimension "d675" = 4
  dimension "d686" = 2
  dimension "d687" = 2
  dimension "d688" = 5
  dimension "d693" = 6
  dimension "d694" = 6
  dimension "d695" = 6
  dimension "d701" = 6
  dimension "d703" = 5
  dimension "d704" = 5
  dimension "d705" = 5
  dimension "d706" = 5
  dimension "d707" = 5
  dimension "d709" = 2
  dimension "d718" = 8.15
  dimension "d719" = 8.15
  dimension "d722" = 2
  dimension "d726" = 9
  dimension "d727" = 9
  dimension "d728" = 9
  dimension "d729" = 5
  dimension "d742" = 2
  dimension "d772" = 5
  dimension "d773" = 2
  dimension "d774" = 2
  dimension "d861" = 3
  dimension "d862" = 3
  dimension "d863" = 3
  dimension "d864" = 3
  dimension "d865" = 3
  dimension "d872" = 2
  dimension "d873" = 2
  dimension "d876" = 5
  dimension "d882" = 2
  dimension "d899" = 17
  dimension "d901" = 34
  dimension "d902" = 2
  dimension "d910" = 5
  dimension "d912" = 5
  dimension "d913" = 5
  dimension "d914" = 5
  dimension "d916" = 2
  dimension "d918" = 3
  dimension "d921" = 2.5
  dimension "d922" = 2.5
  dimension "d923" = 2.5
  dimension "d924" = 2.5
  dimension "d925" = 2
  dimension "d926" = 2
  dimension "d927" = 2
  dimension "d928" = 2.5
  dimension "d929" = 2.5
  dimension "d930" = 2.5
  dimension "d931" = 2.5
  dimension "d932" = 3
  dimension "d933" = 3
  dimension "d934" = 3
  dimension "d935" = 3
  dimension "d936" = 3
  dimension "d937" = 3
  constraint perpendicular L6 L7
  constraint tangent L6 A0
  constraint tangent L6 A1
  constraint tangent L7 A1
  constraint vertical L14
  constraint vertical L8
  constraint horizontal L9
  constraint tangent L8 A2
  constraint tangent L9 A2
  constraint tangent L7 A3
  constraint horizontal L10
  constraint horizontal L11
  constraint horizontal L12
  constraint vertical L13
  constraint coincident L12.start L14
  constraint collinear L14 L15
  constraint tangent L18 A4
  constraint tangent L19 A4
  constraint tangent L18 A5
  constraint equal A4 A5
  constraint horizontal L362
  constraint perpendicular L72 L362
  constraint tangent L72 A29
  constraint tangent L72 A30
  constraint tangent A30 L362
  constraint tangent A23 L362
  constraint horizontal L75
  constraint vertical L79
  constraint tangent L77 A27
  constraint tangent L73 A27
  constraint tangent A24 L77
  constraint equal A24 A27
  constraint tangent L123 A39
  constraint tangent L133 A39
  constraint coincident L111.end L129
  constraint collinear L111 L129
  constraint tangent L110 A40
  constraint tangent L112 A40
  constraint tangent L107 A41
  constraint tangent L131 A41
  constraint equal A40 A41
  constraint concentric A42 A44
  constraint concentric A43 A45
  constraint tangent L137 A44
  constraint tangent L138 A44
  constraint tangent L139 A45
  constraint tangent L140 A45
  constraint tangent L137 A46
  constraint tangent L138 A47
  constraint equal A46 A47
  constraint tangent L139 A48
  constraint equal A46 A48
  constraint tangent L140 A49
  constraint equal A46 A49
  constraint coincident L46 L141.end
  constraint perpendicular L48 L141
  constraint tangent A28 L142
  constraint tangent A21 L143
  constraint tangent A29 L144
  constraint tangent L146 A56
  constraint tangent A56 L298
  constraint tangent L145 A57
  constraint tangent L146 A57
  constraint tangent L147 A58
  constraint tangent L148 A58
  constraint tangent L148 A59
  constraint tangent L147 A60
  constraint tangent L149 A61
  constraint tangent A61 L301
  constraint tangent A62 L301
  constraint tangent L150 A62
  constraint tangent L150 A76
  constraint tangent A76 L303
  constraint tangent A63 A78
  constraint tangent A63 L303
  constraint tangent A70 A73
  constraint tangent A73 A143
  constraint equal A64 A73
  constraint tangent A65 A70
  constraint equal A64 A65
  constraint tangent A66 A67
  constraint equal A64 A66
  constraint collinear L298 L299
  constraint coincident L213.end A73
  constraint concentric A73 A74
  constraint coincident L232 L300.start
  constraint coincident L297.end L301
  constraint collinear L301 L302
  constraint concentric A76 A77
  constraint collinear L303 L304
  constraint equal A88 A89
  constraint tangent A90 L661
  constraint tangent L323 A91
  constraint tangent L324 A91
  constraint tangent A47 L325
  constraint horizontal L325
  constraint tangent A48 L326
  constraint tangent A49 L327
  constraint perpendicular L326 L327
  constraint tangent A46 L328
  constraint tangent L325 A92
  constraint tangent L326 A92
  constraint tangent L327 A93
  constraint tangent L328 A93
  constraint equal A92 A93
  constraint tangent A89 L657
  constraint tangent A89 L659
  constraint tangent A94 L659
  constraint tangent A94 L331
  constraint vertical L329
  constraint tangent A95 L332
  constraint tangent L329 A96
  constraint tangent A96 L657
  constraint tangent L329 A97
  constraint tangent L331 A97
  constraint equal A96 A97
  constraint tangent L330 A98
  constraint equal A96 A98
  constraint tangent L330 A99
  constraint equal A96 A99
  constraint perpendicular L109 L333
  constraint perpendicular L134 L334
  constraint concentric A100 A103
  constraint concentric A101 A102
  constraint tangent L335 A102
  constraint vertical L335
  constraint perpendicular L335 L336
  constraint perpendicular L336 L337
  constraint tangent L339 A103
  constraint perpendicular L336 L339
  constraint perpendicular L339 L340
  constraint tangent L335 A104
  constraint tangent L336 A104
  constraint tangent L339 A105
  constraint tangent L340 A105
  constraint equal A104 A105
  constraint tangent L336 A106
  constraint tangent L337 A106
  constraint tangent L338 A107
  constraint tangent L340 A107
  constraint equal A106 A107
  constraint tangent L339 A108
  constraint tangent A103 A108
  constraint tangent L335 A109
  constraint tangent A102 A109
  constraint equal A108 A109
  constraint tangent L337 A110
  constraint tangent A103 A110
  constraint tangent L338 A111
  constraint tangent A102 A111
  constraint equal A110 A111
  constraint horizontal L341
  constraint vertical L342
  constraint horizontal L343
  constraint vertical L344
  constraint perpendicular L11 L349
  constraint perpendicular L90 L350
  constraint collinear L352 L353
  constraint tangent L352 A112
  constraint tangent L353 A113
  constraint tangent L351 A114
  constraint tangent L351 A115
  constraint perpendicular L354 L357
  constraint perpendicular L354 L355
  constraint perpendicular L356 L357
  constraint collinear L357 L358
  constraint tangent L356 A116
  constraint tangent L357 A116
  constraint tangent L354 A117
  constraint tangent L358 A117
  constraint equal A116 A117
  constraint tangent L355 A118
  constraint tangent L356 A118
  constraint tangent L354 A119
  constraint tangent L355 A119
  constraint equal A118 A119
  constraint collinear L362 L363
  constraint concentric A50 A128
  constraint parallel L366 L367
  constraint tangent L366 A129
  constraint tangent L366 A130
  constraint tangent A128 A130
  constraint tangent L367 A131
  constraint tangent A128 A131
  constraint equal A130 A131
  constraint tangent L367 A132
  constraint equal A130 A132
  constraint concentric A51 A137
  constraint tangent A132 A137
  constraint concentric A85 A138
  constraint tangent A136 A138
  constraint perpendicular L370 L796
  constraint perpendicular L371 L796
  constraint tangent L370 A139
  constraint tangent A137 A139
  constraint tangent A140 L796
  constraint tangent L370 A140
  constraint equal A139 A140
  constraint tangent L371 A141
  constraint tangent A138 A141
  constraint equal A139 A141
  constraint tangent A142 L796
  constraint tangent L371 A142
  constraint equal A139 A142
  constraint concentric A143 A144
  constraint perpendicular L214 L557
  constraint perpendicular L518 L558
  constraint tangent L167 A171
  constraint tangent A144 A171
  constraint tangent A11 L559
  constraint tangent A16 L560
  constraint perpendicular L315 L562
  constraint horizontal L564
  constraint vertical L565
  constraint horizontal L566
  constraint vertical L567
  constraint perpendicular L573 L574
  constraint perpendicular L576 L577
  constraint tangent L576 A174
  constraint tangent L574 A175
  constraint tangent A90 L579
  constraint tangent A36 L580
  constraint perpendicular L114 L581
  constraint coincident A179.centre L593.start
  constraint perpendicular L593 L608
  constraint coincident A178.centre L592.start
  constraint perpendicular L592 L608
  constraint tangent A33 L599
  constraint perpendicular L99 L600
  constraint tangent A31 L602
  constraint vertical L602
  constraint perpendicular L604 L608
  constraint perpendicular L604 L605
  constraint collinear L608 L609
  constraint perpendicular L619 L620
  constraint collinear L623 L624
  constraint perpendicular L576 L634
  constraint perpendicular L577 L635
  constraint perpendicular L576 L636
  constraint perpendicular L577 L637
  constraint perpendicular L640 L641
  constraint perpendicular L641 L642
  constraint perpendicular L642 L643
  constraint vertical L644
  constraint tangent L640 A182
  constraint coincident P13 L641
  constraint coincident P13 L642
  constraint tangent L641 A183
  constraint tangent L642 A183
  constraint coincident P14 L642
  constraint coincident P14 L643
  constraint tangent L642 A184
  constraint tangent L643 A184
  constraint equal A183 A184
  constraint tangent L643 A185
  constraint tangent L644 A185
  constraint equal A183 A185
  constraint tangent L644 A186
  constraint tangent A182 A186
  constraint tangent A191 L653
  constraint parallel L652 L653
  constraint perpendicular L652 L654
  constraint tangent L653 A194
  constraint tangent L654 A194
  constraint tangent L652 A195
  constraint tangent L654 A195
  constraint equal A194 A195
  constraint tangent A98 L655
  constraint tangent A99 L656
  constraint concentric A86 A203
  constraint concentric A87 A196
  constraint collinear L657 L658
  constraint concentric A196 A197
  constraint collinear L659 L660
  constraint collinear L661 L662
  constraint concentric A203 A204
  constraint tangent L658 A205
  constraint tangent A203 A205
  constraint tangent L663 A206
  constraint tangent A204 A206
  constraint equal A205 A206
  constraint tangent L668 A207
  constraint tangent A204 A207
  constraint equal A205 A207
  constraint tangent L657 A208
  constraint tangent A203 A208
  constraint equal A205 A208
  constraint tangent A201 A209
  constraint tangent L667 A209
  constraint equal A205 A209
  constraint tangent L666 A210
  constraint tangent A201 A210
  constraint equal A205 A210
  constraint tangent A196 A211
  constraint tangent L659 A211
  constraint equal A205 A211
  constraint tangent A196 A212
  constraint tangent L660 A212
  constraint equal A205 A212
  constraint tangent A197 A213
  constraint tangent L661 A213
  constraint equal A205 A213
  constraint tangent A197 A214
  constraint tangent L662 A214
  constraint equal A205 A214
  constraint tangent A172 A224
  constraint tangent A221 A224
  constraint tangent A173 A225
  constraint tangent A222 A225
  constraint concentric A223 A226
  constraint concentric A226 A227
  constraint tangent A221 A228
  constraint tangent A227 A228
  constraint tangent A222 A229
  constraint tangent A227 A229
  constraint equal A228 A229
  constraint tangent A187 L674
  constraint tangent A188 L675
  constraint collinear L676 L677
  constraint tangent L674 A230
  constraint tangent L676 A230
  constraint tangent L675 A231
  constraint tangent L677 A231
  constraint equal A230 A231
  constraint collinear L678 L679
  constraint tangent L679 A232
  constraint tangent L678 A233
  constraint equal A232 A233
  constraint perpendicular L676 L713
  constraint tangent A277 L897
  constraint parallel L318 L747
  constraint parallel L319 L750
  constraint tangent L749 A283
  constraint tangent L748 A283
  constraint tangent L748 A284
  constraint tangent A284 L750
  constraint equal A283 A284
  constraint tangent A285 L750
  constraint tangent L747 A285
  constraint equal A283 A285
  constraint tangent L747 A286
  constraint equal A283 A286
  constraint coincident L481 L749.end
  constraint coincident L444 L452.end
  constraint collinear L750 L751
  constraint coincident A285 L452.start
  constraint coincident L381.end A286
  constraint concentric A286 A287
  constraint horizontal L787
  constraint tangent L788 A300
  constraint tangent L791 A300
  constraint tangent L790 A301
  constraint tangent L791 A301
  constraint equal A300 A301
  constraint tangent L789 A302
  constraint tangent L790 A302
  constraint equal A300 A302
  constraint tangent L788 A303
  constraint tangent L789 A303
  constraint equal A300 A303
  constraint concentric A273 A308
  constraint collinear L796 L797
  constraint collinear L797 L798
  constraint collinear L798 L799
  constraint tangent A308 A311
  constraint tangent L796 A311
  constraint tangent A308 A312
  constraint tangent L797 A312
  constraint equal A311 A312
  constraint tangent L797 A313
  constraint tangent A309 A313
  constraint equal A311 A313
  constraint tangent A309 A314
  constraint tangent L798 A314
  constraint equal A311 A314
  constraint tangent L798 A315
  constraint tangent A310 A315
  constraint equal A311 A315
  constraint tangent L799 A316
  constraint tangent A310 A316
  constraint equal A311 A316
  constraint coincident L524.end L800
  constraint collinear L800 L801
  constraint tangent A317 L802
  constraint tangent A318 L803
  constraint tangent L802 A318
  constraint tangent L803 A319
  constraint tangent L804 A321
  constraint tangent L804 A320
  constraint tangent A7 L831
  constraint tangent A20 L832
  constraint tangent A0 L833
  constraint tangent A15 L834
  constraint tangent A5 L835
  constraint tangent A8 L836
  constraint tangent A319 L838
  constraint parallel L837 L838
  constraint perpendicular L837 L839
  constraint tangent A317 L840
  constraint tangent L838 A348
  constraint tangent L839 A348
  constraint tangent L837 A349
  constraint tangent L839 A349
  constraint equal A348 A349
  constraint tangent L837 A350
  constraint tangent L840 A350
  constraint equal A348 A350
  constraint perpendicular L119 L859
  constraint horizontal L865
  constraint horizontal L866
  constraint coincident A10.centre L866.start
  constraint vertical L867
  constraint vertical L868
  constraint concentric A369 A370
  constraint tangent A370 A371
  constraint tangent A296 A371
  constraint tangent A295 A372
  constraint tangent A370 A372
  constraint equal A371 A372
  constraint perpendicular L143 L881
  constraint perpendicular L881 L882
  constraint parallel L881 L883
  constraint tangent L881 A381
  constraint tangent L882 A381
  constraint tangent L882 A382
  constraint tangent L883 A382
  constraint equal A381 A382
  constraint tangent A320 L885
  constraint tangent A379 L886
  constraint perpendicular L805 L894
  constraint perpendicular L142 L895
  constraint perpendicular L895 L896
  constraint tangent L894 A389
  constraint tangent L896 A389
  constraint tangent L895 A390
  constraint tangent L896 A390
  constraint equal A389 A390
  constraint concentric A276 A391
  constraint tangent A391 A392
  constraint tangent L897 A392
  constraint tangent A391 A393
  constraint tangent A277 A393
  constraint tangent A236 L898
  constraint tangent A126 L900
  constraint tangent A237 L901
  constraint tangent A246 L902
  constraint tangent A245 L904
  constraint tangent A327 L906
  constraint tangent A253 L907
  constraint tangent A256 L908
  constraint tangent A112 L910
  constraint tangent A232 L911
  constraint tangent A233 L912
  constraint tangent A113 L913
  constraint horizontal L917
  constraint vertical L918
  constraint horizontal L915
  constraint vertical L914
  constraint concentric A394 A399
  constraint concentric A396 A398
  constraint concentric A397 A401
  constraint concentric A395 A400
  constraint coincident A396 L916.start
  constraint collinear L915 L916
  constraint tangent L914 A402
  constraint tangent A399 A402
  constraint tangent A399 A403
  constraint tangent L917 A403
  constraint equal A402 A403
  constraint tangent L914 A404
  constraint tangent A398 A404
  constraint equal A402 A404
  constraint tangent L915 A405
  constraint tangent A398 A405
  constraint equal A402 A405
  constraint tangent L915 A406
  constraint tangent A401 A406
  constraint equal A402 A406
  constraint tangent L918 A407
  constraint tangent A401 A407
  constraint equal A402 A407
  constraint tangent A400 A408
  constraint tangent L918 A408
  constraint equal A402 A408
  constraint tangent A400 A409
  constraint tangent L917 A409
  constraint equal A402 A409
  constraint concentric A410 A412
  constraint tangent L919 A413
  constraint tangent A412 A414
  constraint tangent L920 A414
  constraint equal A413 A414
  constraint tangent A412 A415
  constraint tangent L919 A415
  constraint equal A413 A415
  constraint tangent L921 A417
  constraint tangent L922 A417
  constraint parallel L921 L922
  constraint perpendicular L342 L923
  constraint perpendicular L923 L924
  constraint perpendicular L924 L925
  constraint perpendicular L923 L926
  constraint horizontal L931
  constraint coincident P15 L923